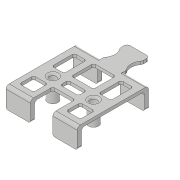
# Autodesk Inventor part: Robot_Stand
Saved by Autodesk Inventor 2019 (Build 230136000, 136)
## iProperties
Created: 2023-04-04
Part Number: Robot_Stand
Material: Generic
Document SubType Name: Modeling
Designer: Oudenas
Density: 1 g/cm^3
Appearance: Default
Author: Oudenas
Autodesk Inventor part; units mm, degrees
ref_plane "YZ Plane" through (0, 0, 0) normal (1, 0, 0) x (0, 1, 0)
ref_plane "XZ Plane" through (0, 0, 0) normal (0, 1, 0) x (-1, 0, 0)
ref_plane "XY Plane" through (0, 0, 0) normal (0, 0, 1) x (1, 0, 0)
sketch "Sketch1" plane through (0, 0, 0) normal (0, 1, 0) x (-1, 0, 0)
  line L0 (35, 35) -> (-35, 35)
  line L1 (-35, 35) -> (-35, -35)
  line L2 (-35, -35) -> (35, -35)
  line L3 (35, -35) -> (35, 35)
  line L4 (35, 35) -> (-35, -35) construction
  line L5 (-35, 35) -> (35, -35) construction
  line L6 (11, -35) -> (-11, -35)
  line L7 (-11, -35) -> (-11, -37.0627)
  line L8 (-11, -60) -> (11, -60)
  line L9 (11, -60) -> (11, -52.9373)
  line L10 (11, -35) -> (-11, -60) construction
  line L11 (-11, -35) -> (11, -60) construction
  circle A0 centre (-20, -45) radius 12
  circle A1 centre (20, -45) radius 12
  line L12 (-11, -37.0627) -> (-11, -52.9373)
  line L13 (-11, -52.9373) -> (-11, -60)
  line L14 (0, -47.5) -> (0, -35) construction
  line L15 (11, -37.0627) -> (11, -35)
  line L16 (11, -52.9373) -> (11, -37.0627)
  point P0 (0, 0)
  point P1 (0, -47.5)
  point P2 (0, 0)
  dimension "d0" = 70
  dimension "d1" = 70
  dimension "d58" = 22
  dimension "d59" = 25
  dimension "d64" = 24
  dimension "d66" = 24
  dimension "d68" = 10
  dimension "d69" = 10
  dimension "d70" = 20
  dimension "d71" = 20
  constraints: 34 end point, 12 parallel, 7 midpoint, 4 perpendicular, 4 point on circle, 2 centre point, 2 horizontal, 1 collinear, 1 vertical alignment
  measures "d0" distance of L2.end L1.end
  measures "d1" distance of L1.end L0.end
  measures "d58" distance of L8.end L8.start
  measures "d59" distance of L8.start L6.end
  measures "d64" diameter of A0
  measures "d66" diameter of A1
  measures "d68" distance from line of L2 A1.centre
  measures "d69" distance from line of A0.centre L2
  measures "d70" distance from line of A1.centre L14
  measures "d71" horizontal distance of point (0, -47.5) A0.centre
extrude "Extrusion1" add sketch "Sketch1" along normal blind 3 contours L3 L2 A1 A0 L1 L0 | L2 A1 | A0 L2 | A0 L7 L2 L15 A1 L9 L8 L13
sketch "Sketch2" plane through (0, 3, 0) normal (0, 1, 0) x (1, 0, 0)
  line L0 (-11, -13) -> (11, -13)
  line L1 (11, -13) -> (11, -35)
  line L2 (11, -35) -> (-11, -35)
  line L3 (-11, -35) -> (-11, -13)
  line L4 (-11, -13) -> (11, -35) construction
  line L5 (11, -13) -> (-11, -35) construction
  line L6 (-35, -35) -> (35, -35) projected
  point P0 (0, 0)
  point P1 (0, -24)
  point P2 (0, -24)
  dimension "d4" = 22
  dimension "d5" = 22
  constraints: 12 end point, 3 midpoint, 2 parallel, 1 collinear, 1 horizontal, 1 perpendicular, 1 vertical alignment
  measures "d4" distance of L1.end L2.end
  measures "d5" distance of L0.end L1.end
extrude "Extrusion2" cut sketch "Sketch2" against normal blind 20
sketch "Sketch3" plane through (0, 3, 0) normal (0, 1, 0) x (1, 0, 0)
  line L0 (11, 5) -> (-11, 5)
  line L1 (-11, 5) -> (-11, 27)
  line L2 (-11, 27) -> (11, 27)
  line L3 (11, 27) -> (11, 5)
  line L4 (11, 5) -> (-11, 27) construction
  line L5 (-11, 5) -> (11, 27) construction
  line L6 (35, 35) -> (-35, 35) projected
  point P0 (0, 0)
  point P1 (0, 16)
  point P2 (0, 16)
  dimension "d9" = 22
  dimension "d52" = 8
  constraints: 12 end point, 3 midpoint, 2 parallel, 1 horizontal, 1 perpendicular, 1 vertical alignment
  measures "d9" distance of L0.end L1.end
  measures "d52" distance between parallel lines of L2 L6
extrude "Extrusion3" cut sketch "Sketch3" against normal blind 20
sketch "Sketch4" plane through (0, 0, 0) normal (0, -1, 0) x (1, 0, 0)
  line L0 (-35, -35) -> (-35, 35) projected
  line L1 (-11, 35) -> (-11, 13) projected
  line L2 (11, 13) -> (11, 35) projected
  line L3 (35, 35) -> (35, -35) projected
  line L4 (-11, -5) -> (-11, -27) projected
  line L5 (-11, 13) -> (11, 13) construction
  line L6 (0, 13) -> (0, -5) construction
  line L7 (-11, -5) -> (11, -5) construction
  line L8 (-35, 4) -> (35, 4) construction
  circle A0 centre (-20, 4) radius 5
  circle A1 centre (20, 4) radius 5
  line L9 (-35, 35) -> (-11, 35)
  line L10 (-11, 35) -> (-11, 31)
  line L11 (-11, 31) -> (-35, 31)
  line L12 (-35, 31) -> (-35, 35)
  line L13 (11, 35) -> (11, 13) projected
  line L14 (11, 35) -> (35, 35)
  line L15 (35, 35) -> (35, 31)
  line L16 (35, 31) -> (11, 31)
  line L17 (11, 31) -> (11, 35)
  line L18 (35, -35) -> (11, -35)
  line L19 (11, -35) -> (11, -31)
  line L20 (11, -31) -> (35, -31)
  line L21 (35, -31) -> (35, -35)
  line L22 (-35, -35) -> (-11, -35)
  line L23 (-11, -35) -> (-11, -31)
  line L24 (-11, -31) -> (-35, -31)
  line L25 (-35, -31) -> (-35, -35)
  point P0 (0, 0)
  dimension "d18" = 4
  dimension "d19" = 10
  dimension "d20" = 10
  dimension "d21" = 15
  dimension "d22" = 15
  dimension "d54" = 4
  dimension "d55" = 4
  dimension "d60" = 24
  dimension "d61" = 4
  dimension "d62" = 24
  dimension "d63" = 4
  constraints: 36 end point, 8 parallel, 6 point on line, 5 perpendicular, 4 horizontal, 2 centre point, 2 midpoint
  measures "d18" distance from line of L8 point (0, 0)
  measures "d19" diameter of A0
  measures "d20" diameter of A1
  measures "d21" distance from line of A0.centre L0
  measures "d22" distance from line of L3 A1.centre
  measures "d54" distance between parallel lines of L11 L9
  measures "d55" distance between parallel lines of L16 L14
  measures "d60" distance of L0.start L22.end
  measures "d61" distance between parallel lines of L22 L24
  measures "d62" distance of L3.end L18.end
  measures "d63" distance between parallel lines of L20 L18
extrude "Extrusion4" add sketch "Sketch4" along normal blind 17
sketch "Sketch7" plane through (20, -17, 4) normal (0, -1, 0) x (1, 0, 0)
  circle A0 centre (0, 0) radius 5 projected
  circle A1 centre (0, 0) radius 3.5
  circle A2 centre (-40, 0) radius 5 projected
  circle A3 centre (-40, 0) radius 3.5
  point P0 (-20, -4)
  dimension "d31" = 7
  dimension "d32" = 7
  constraints: 2 centre point, 2 coincident
  measures "d31" diameter of A1
  measures "d32" diameter of A3
extrude "Extrusion6" cut sketch "Sketch7" against normal blind 20 contours A1 | A3
sketch "Sketch8" plane through (0, 0, 0) normal (0, -1, 0) x (1, 0, 0)
  line L0 (-35, 35) -> (-11, 35) construction
  line L1 (35, -35) -> (-35, -35) construction
  line L2 (35, -35) -> (-35, -35) construction
  line L3 (11, 35) -> (35, 35) construction
  line L4 (-29, -4) -> (-17, -4)
  line L5 (-17, -4) -> (-17, -26)
  line L6 (-17, -26) -> (-29, -26)
  line L7 (-29, -26) -> (-29, -4)
  line L8 (-29, -4) -> (-17, -26) construction
  line L9 (-17, -4) -> (-29, -26) construction
  line L10 (17, -26) -> (29, -26)
  line L11 (29, -26) -> (29, -4)
  line L12 (29, -4) -> (17, -4)
  line L13 (17, -4) -> (17, -26)
  line L14 (17, -26) -> (29, -4) construction
  line L15 (29, -26) -> (17, -4) construction
  line L16 (-30, 13) -> (-16, 13)
  line L17 (-16, 13) -> (-16, 27)
  line L18 (-16, 27) -> (-30, 27)
  line L19 (-30, 27) -> (-30, 13)
  line L20 (-30, 13) -> (-16, 27) construction
  line L21 (-16, 13) -> (-30, 27) construction
  line L22 (16, 27) -> (30, 27)
  line L23 (30, 27) -> (30, 13)
  line L24 (30, 13) -> (16, 13)
  line L25 (16, 13) -> (16, 27)
  line L26 (16, 27) -> (30, 13) construction
  line L27 (30, 27) -> (16, 13) construction
  circle A0 centre (20, 4) radius 3.5 projected
  circle A1 centre (-20, 4) radius 3.5 projected
  line L28 (20, 4) -> (-20, 4) construction
  line L29 (-9, 0) -> (9, 0)
  line L30 (9, 0) -> (9, 8)
  line L31 (9, 8) -> (-9, 8)
  line L32 (-9, 8) -> (-9, 0)
  line L33 (-9, 0) -> (9, 8) construction
  line L34 (9, 0) -> (-9, 8) construction
  line L35 (23, 35) -> (23, -35) construction
  line L36 (-23, 35) -> (-23, -35) construction
  point P0 (0, 0)
  point P1 (-23, -15)
  point P2 (23, -15)
  point P3 (-23, 20)
  point P4 (23, 20)
  point P5 (0, 4)
  point P6 (-23, 20)
  point P7 (-23, 20)
  point P8 (-23, -15)
  point P9 (23, -15)
  point P10 (23, 20)
  dimension "d35" = 12
  dimension "d36" = 22
  dimension "d37" = 12
  dimension "d38" = 22
  dimension "d39" = 20
  dimension "d40" = 20
  dimension "d41" = 14
  dimension "d42" = 14
  dimension "d43" = 14
  dimension "d44" = 14
  dimension "d45" = 15
  dimension "d46" = 15
  dimension "d56" = 18
  dimension "d57" = 8
  constraints: 66 end point, 18 midpoint, 10 parallel, 7 perpendicular, 6 horizontal, 6 point on line
  measures "d35" distance of L5.end L6.end
  measures "d36" distance of L4.end L5.end
  measures "d37" distance of L12.end L11.end
  measures "d38" distance of L11.end L10.end
  measures "d39" distance from line of point (-23, -15) L1
  measures "d40" distance from line of L2 point (23, -15)
  measures "d41" distance of L18.end L17.end
  measures "d42" distance of L17.end L16.end
  measures "d43" distance of L23.end L24.end
  measures "d44" distance of L22.end L23.end
  measures "d45" distance from line of L3 point (23, 20)
  measures "d46" distance from line of point (-23, 20) L0
  measures "d56" distance of L31.end L30.end
  measures "d57" distance of L30.end L29.end
extrude "Extrusion7" cut sketch "Sketch8" against normal blind 3 contours L4 L5 L6 L7 | L13 L12 L11 L10 | L19 L18 L17 L16 | L22 L23 L24 L25 | L32 L31 L30 L29
fillet "Fillet2" radius 3 19 edges at (-25, 0, 4) (15, 0, 4) (23, 3, 35) (-23, 3, 35) (-23, 0, 31) (23, 0, 31) (11, 1.5, -35) (-23, 3, -35) (23, 3, -35) (-23, 0, -31) (23, 0, -31) (11, 1.5, -60) (-11, 1.5, -60) (-11, 1.5, -52.9373) (-11, 1.5, -37.0627) (11, 1.5, -37.0627) (11, 1.5, -52.9373) (-11, 0, -33) (11, 0, -33)
fillet "Fillet3" radius 2 36 edges at (29, 1.5, -26) (17, 1.5, -26) (29, 1.5, -4) (17, 1.5, -4) (16, 1.5, 27) (30, 1.5, 27) (16, 1.5, 13) (30, 1.5, 13) (-30, 1.5, 13) (-30, 1.5, 27) (-16, 1.5, 27) (-16, 1.5, 13) (-17, 1.5, -26) (-17, 1.5, -4) (-29, 1.5, -4) (-29, 1.5, -26) (-11, 1.5, -5) (11, 1.5, -5) (11, 1.5, 13) (-11, 1.5, 13) (16.5, 3, 4) (-23.5, 3, 4) (11, 1.5, -27) (-11, 1.5, -27) (-9, 1.5, 8) (-9, 1.5, 0) (9, 1.5, 0) (9, 1.5, 8) (-11, -17, 33) (-35, -17, 33) (11, -17, 33) (35, -17, 33) (11, -17, -33) (-35, -17, -33) (-11, -17, -33) (35, -17, -33)
equation "\"d55\" = d54"
equation "\"d40\" = d39"
equation "\"d46\" = d45"
body "Solid1"
